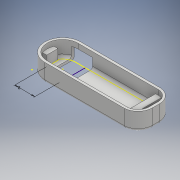
# Autodesk Inventor part: bottom
Saved by Autodesk Inventor 2017 (Build 210142000, 142)
## iProperties
Part Number: bottom
Material: Типовые
Document SubType Name: Modeling
Designer: roman
Density: 1 g/cm^3
Appearance: По умолчанию
Author: roman
Autodesk Inventor part; units mm, degrees
ref_plane "YZ Plane" through (0, 0, 0) normal (1, 0, 0) x (0, 1, 0)
ref_plane "XZ Plane" through (0, 0, 0) normal (0, 1, 0) x (-1, 0, 0)
ref_plane "XY Plane" through (0, 0, 0) normal (0, 0, 1) x (1, 0, 0)
sketch "Эскиз1" plane through (0, 0, 0) normal (0, 0, 1) x (1, 0, 0)
  arc A0 (6.1718, 12.1916) -> (6.0205, -0.0083) centre (6, 6.0928) ccw
  line L0 (6.1718, 12.1916) -> (6.0205, -0.0083) construction
  line L1 (6.1718, 12.1916) -> (18.3727, 12.1916) construction
  arc A1 (42.148, 8.0153) -> (37.9718, 12.1916) centre (37.9718, 8.0153) ccw
  arc A2 (37.8204, -0.0083) -> (42.148, 4.3193) centre (37.8204, 4.3193) ccw
  arc A3 (6.1001, 13.1916) -> (6.1001, -1.0083) centre (6.1001, 6.0916) ccw
  arc A4 (43.148, 7.5237) -> (37.78, 13.1916) centre (37.4718, 7.5237) ccw
  arc A5 (37.7733, -1.0083) -> (43.148, 4.6599) centre (37.4718, 4.6599) ccw
  line L2 (6.1718, 12.1916) -> (37.9718, 12.1916)
  line L3 (37.78, 13.1916) -> (6.1001, 13.1916)
  line L4 (6.0205, -0.0083) -> (37.8204, -0.0083)
  line L5 (37.7733, -1.0083) -> (6.1001, -1.0083)
  line L6 (42.148, 8.0153) -> (42.148, 4.3193)
  line L7 (43.148, 7.5237) -> (43.148, 4.6599)
  point P0 (0, 0)
  point P1 (0, 0)
  dimension "d7" = 1.5
  dimension "d0" = 90.71
  dimension "d1" = 4.1763
  dimension "d2" = 5.6763
  dimension "d3" = 5.6763
  dimension "d4" = 1
  dimension "d5" = 1
  dimension "d8" = 12.1999
  dimension "d9" = 31.8
  dimension "d10" = 31.7998
  dimension "d13" = 1
  constraints: 16 end point, 12 point on circle, 6 centre point, 6 tangent, 2 horizontal, 2 parallel, 2 vertical, 1 equal length
  measures "d0" angle of L0 L1
  measures "d1" radius of A1
  measures "d2" radius of A4
  measures "d3" radius of A5
  measures "d4" distance between parallel lines of L2 L3
  measures "d5" distance between parallel lines of L5 L4
  measures "d8" distance between parallel lines of L4 L2
  measures "d9" distance of L0.start L2.end
  measures "d10" distance of L4.start L4.end
  measures "d13" distance between parallel lines of L7 L6
extrude "main_walls" add sketch "Эскиз1" along normal blind 6
sketch "Эскиз2" plane through (0, 0, 0) normal (0, 0, -1) x (-1, 0, 0)
  line L0 (-37.7733, -1.0083) -> (-6.1001, -1.0083) projected
  arc A0 (-6.1001, -1.0083) -> (-6.1001, 13.1916) centre (-6.1001, 6.0916) ccw projected
  line L1 (-6.1001, 13.1916) -> (-37.78, 13.1916) projected
  arc A1 (-37.78, 13.1916) -> (-43.148, 7.5237) centre (-37.4718, 7.5237) ccw projected
  line L2 (-43.148, 7.5237) -> (-43.148, 4.6599) projected
  arc A2 (-43.148, 4.6599) -> (-37.7733, -1.0083) centre (-37.4718, 4.6599) ccw projected
  point P0 (0, 0)
extrude "floor" add sketch "Эскиз2" along normal blind 1
sketch "Эскиз3" plane through (0, 0, 0) normal (0, 0, 1) x (1, 0, 0)
  line L0 (42.148, 4.3193) -> (42.148, 8.0153) projected
  arc A0 (42.148, 8.0153) -> (37.9718, 12.1916) centre (37.9718, 8.0153) ccw projected
  line L1 (37.9718, 12.1916) -> (6.1718, 12.1916) projected
  arc A1 (6.1718, 12.1916) -> (6.0205, -0.0083) centre (6, 6.0928) ccw projected
  line L2 (6.0205, -0.0083) -> (37.8204, -0.0083) projected
  arc A2 (37.8204, -0.0083) -> (42.148, 4.3193) centre (37.8204, 4.3193) ccw projected
  line L3 (-0.1012, 8.3416) -> (1.8988, 8.3416)
  line L4 (1.8988, 8.3416) -> (1.8988, 3.8416)
  line L5 (1.8988, 3.8416) -> (-0.1012, 3.8416)
  line L6 (-0.1012, 3.8416) -> (-0.1012, 8.3416)
  arc A3 (6.1718, 12.1916) -> (6.0205, -0.0083) centre (6, 6.0928) ccw projected
  arc A4 (42.148, 8.0153) -> (37.9718, 12.1916) centre (37.9718, 8.0153) ccw projected
  line L7 (6.1718, 12.1916) -> (37.9718, 12.1916) projected
  arc A5 (37.8204, -0.0083) -> (42.148, 4.3193) centre (37.8204, 4.3193) ccw projected
  line L8 (6.0205, -0.0083) -> (37.8204, -0.0083) projected
  line L9 (36.948, 12.1916) -> (39.448, 12.1916)
  line L10 (39.448, 12.1916) -> (39.448, -0.0083)
  line L11 (39.448, -0.0083) -> (36.948, -0.0083)
  line L12 (36.948, -0.0083) -> (36.948, 12.1916)
  point P0 (0, 0)
  dimension "d16" = 2
  dimension "d17" = 4.5
  dimension "d18" = 12.1999
  dimension "d19" = 3.85
  dimension "d22" = 2.7
  dimension "d23" = 2.5
  constraints: 16 end point, 4 parallel, 2 horizontal, 2 perpendicular, 2 point on line, 1 tangent
  measures "d16" distance of L4.end L5.end
  measures "d17" distance of L3.end L4.end
  measures "d18" distance between parallel lines of L2 L1
  measures "d19" distance between parallel lines of L2 L5
  measures "d22" distance between parallel lines of L0 L10
  measures "d23" distance between parallel lines of L10 L12
extrude "supports" add sketch "Эскиз3" along normal blind 4 contours L10 L11 A2 | A2 L2 L12 L1 A0 L10 | A0 L9 L10 | L5 L6 A1 | A1 L3 L4 L5 | A1 L6 L3
fillet "bottom_rounding" radius 1 13 edges at (21.5599, 12.1916, 0) (21.4843, -0.0083, 0) (2.5814, 1.0393, 0) (2.6433, 11.1876, 0) (42.148, 6.1673, 0) (41.4101, 1.9022, 0) (41.4073, 10.3898, 0) (-0.9999, 6.0916, -1) (21.94, 13.1916, -1) (21.9367, -1.0083, -1) (43.148, 6.0918, -1) (41.593, 11.4269, -1) (41.5907, 0.7543, -1)
sketch "Эскиз5" plane through (0, 0, 0) normal (0, 0, 1) x (1, 0, 0)
  arc A0 (1.4224, 3.8416) -> (6.0188, 0.9917) centre (6, 6.0928) ccw projected
  line L0 (36.948, 0.9917) -> (6.0188, 0.9917) projected
  line L1 (36.948, 0.9917) -> (36.948, 11.1916) projected
  line L2 (6.1571, 11.1916) -> (36.948, 11.1916) projected
  arc A1 (6.1571, 11.1916) -> (1.4212, 8.3416) centre (6, 6.0928) ccw projected
  line L3 (1.4212, 8.3416) -> (1.8988, 8.3416) projected
  line L4 (1.8988, 8.3416) -> (1.8988, 3.8416) projected
  line L5 (1.8988, 3.8416) -> (1.4224, 3.8416) projected
  line L6 (9.8988, 0.9917) -> (9.8988, 11.1916)
  point P0 (0, 0)
  dimension "d27" = 8
  constraints: 2 end point, 2 point on line, 1 vertical
  measures "d27" distance between parallel lines of L6 L4
sketch "Эскиз6" plane through (0, 0, -1) normal (0, 0, -1) x (-1, 0, 0)
  line L0 (-1.8988, 8.3416) -> (-1.8988, 3.8416) projected
  line L1 (-1.4212, 8.3416) -> (-1.8988, 8.3416) projected
  arc A0 (-1.4212, 8.3416) -> (-6.1571, 11.1916) centre (-6, 6.0928) ccw projected
  line L2 (-1.8988, 3.8416) -> (-1.4224, 3.8416) projected
  arc A1 (-6.0188, 0.9917) -> (-1.4224, 3.8416) centre (-6, 6.0928) ccw projected
  line L3 (-6.1001, -0.0083) -> (-37.7455, -0.0083) projected
  arc A2 (-6.1001, -0.0083) -> (-6.1001, 12.1916) centre (-6.1001, 6.0916) ccw projected
  line L4 (-37.7515, 12.1916) -> (-6.1001, 12.1916) projected
  arc A3 (-37.7515, 12.1916) -> (-42.148, 7.5237) centre (-37.4718, 7.5237) ccw projected
  line L5 (-42.148, 4.6599) -> (-42.148, 7.5237) projected
  arc A4 (-42.148, 4.6599) -> (-37.7455, -0.0083) centre (-37.4718, 4.6599) ccw projected
  line L6 (-6.1571, 11.1916) -> (-36.948, 11.1916) projected
  line L7 (-36.948, 0.9917) -> (-6.0188, 0.9917) projected
  line L8 (-11.8741, 11.1916) -> (-11.8741, 0.9917)
  line L9 (-3.8741, 10.7299) -> (-3.8741, 1.4557)
  line L10 (-6.1001, 13.1916) -> (-37.78, 13.1916) projected
  line L11 (-3.8741, 10.7299) -> (-11.8741, 10.7299)
  line L12 (-11.8741, 10.7299) -> (-11.8741, 13.1916)
  line L13 (-11.8741, 13.1916) -> (-3.8741, 13.1916)
  line L14 (-3.8741, 13.1916) -> (-3.8741, 10.7299)
  point P0 (0, 0)
  dimension "d31" = 8
  constraints: 12 end point, 3 point on line, 2 parallel, 2 perpendicular, 2 point on circle, 1 horizontal, 1 vertical
  measures "d31" distance between parallel lines of L9 L8
extrude "Выдавливание5" cut sketch "Эскиз6" against normal blind 5 contours L11 L8 L6 A0 | L9 A1 L7 L8 L11 | A0 L6 L12 L4 A2 L14 | A2 L4 L12 L10 L13 L14
equation "\"d2\" = d1 + d7"
equation "\"d3\" = d1 + d7"
equation "\"d5\" = d4"
equation "\"d13\" = d4"
equation "\"d19\" = -0.5 * d17 + 0.5 * d18"
